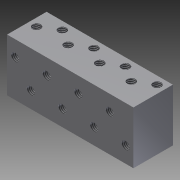
# Autodesk Inventor part: t-manifold ems
Saved by Autodesk Inventor 2011 (Build 150239000, 239)
## iProperties
Created: 2012-03-13
Part Number: t-manifold ems
Document SubType Name: Modeling
Designer: Marc
Density: 1 g/cm^3
Author: Marc
Autodesk Inventor part; units mm, degrees
ref_plane "YZ Plane" through (0, 0, 0) normal (1, 0, 0) x (0, 1, 0)
sketch "Sketch1" plane through (0, 0, 0) normal (0, 0, 1) x (1, 0, 0)
  line L0 (0, 25.4) -> (60.96, 25.4)
  line L1 (60.96, 25.4) -> (60.96, 0)
  line L2 (60.96, 0) -> (0, 0)
  line L3 (0, 0) -> (0, 25.4)
  dimension "tmanifold_width" = 60.96
  dimension "tmanifold_depth" = 25.4
  constraints: 8 end point, 2 parallel, 1 coincident, 1 horizontal, 1 perpendicular
  measures "tmanifold_width" distance of L1.end L2.end
  measures "tmanifold_depth" distance of L0.end L1.end
extrude "Extrusion1" add sketch "Sketch1" along normal blind 19.05
sketch "Sketch2" plane through (0, 0, 19.05) normal (0, 0, 1) x (1, 0, 0)
  line L0 (60.96, 25.4) -> (60.96, 0) projected
  line L1 (0, 25.4) -> (60.96, 25.4) projected
  line L2 (0, 0) -> (0, 25.4) projected
  line L3 (0, 12.7) -> (60.96, 12.7) construction
  line L4 (3.81, 17.78) -> (3.81, 12.7) construction
  line L5 (11.43, 7.62) -> (11.43, 12.7) construction
  point P0 (19.05, 17.78)
  point P1 (26.67, 7.62)
  point P2 (34.29, 17.78)
  point P3 (41.91, 7.62)
  point P4 (49.53, 17.78)
  point P5 (57.15, 7.62)
  dimension "d5" = 7.62
  dimension "d6" = 7.62
  dimension "d9" = 15.24
  dimension "d14" = 3.81
  constraints: 6 end point, 2 midpoint, 2 perpendicular, 2 point on line, 1 horizontal, 1 parallel, 6 other
  measures "d5" horizontal distance of L5.start L4.start
  measures "d6" distance from line of L1 L4.start
  measures "d9" distance of L5.start point (26.67, 7.62)
  measures "d14" distance from line of L2 L4.start
hole "top 10-32 ports" at (3.81, 17.78, 19.05) at (11.43, 7.62, 19.05) at (26.67, 7.62, 19.05) at (19.05, 17.78, 19.05) at (41.91, 7.62, 19.05) at (34.29, 17.78, 19.05) at (57.15, 7.62, 19.05) at (49.53, 17.78, 19.05) direction (0, 0, -1) diameter 3.9624 depth 6.604 thread size "10-32 UNF" class "2B" standard "ANSI Unified Screw Threads"
sketch "Sketch3" plane through (0, 0, 0) normal (0, -1, 0) x (1, 0, 0)
  line L0 (60.96, 19.05) -> (0, 19.05) projected
  line L1 (60.96, 0) -> (0, 0) projected
  line L2 (1.8288, 12.446) -> (1.8288, 19.05) projected
  line L3 (5.7912, 12.446) -> (5.7912, 19.05) projected
  line L4 (5.7912, 12.446) -> (1.8288, 12.446) projected
  line L5 (9.4488, 12.446) -> (9.4488, 19.05) projected
  line L6 (13.4112, 12.446) -> (13.4112, 19.05) projected
  line L7 (13.4112, 12.446) -> (9.4488, 12.446) projected
  line L8 (3.81, 12.446) -> (3.81, 0) construction
  line L9 (11.43, 12.446) -> (11.43, 0) construction
  circle A0 centre (3.81, 8.636) radius 3.81 construction
  circle A1 centre (11.43, 3.81) radius 3.81 construction
  point P0 (19.05, 8.636)
  point P1 (26.67, 3.81)
  point P2 (34.29, 8.636)
  point P3 (41.91, 3.81)
  point P4 (49.53, 8.636)
  point P5 (57.15, 3.81)
  dimension "d22" = 7.62
  dimension "d25" = 15.24
  dimension "d78" = 8.636
  dimension "d79" = 3.81
  constraints: 4 end point, 4 point on line, 2 centre point, 2 coincident, 2 midpoint, 2 perpendicular, 2 tangent, 1 equal radius, 1 horizontal, 6 other
  measures "d22" diameter of A0
  measures "d25" distance of point (3.81, 8.636) point (19.05, 8.636)
  measures "d78" distance from line of L1 point (49.53, 8.636)
  measures "d79" distance from line of L1 point (57.15, 3.81)
hole "front 10-32 ports" at (3.81, 0, 8.636) at (11.43, 0, 3.81) at (19.05, 0, 8.636) at (26.67, 0, 3.81) at (34.29, 0, 8.636) at (41.91, 0, 3.81) at (49.53, 0, 8.636) at (57.15, 0, 3.81) direction (0, 1, 0) diameter 3.9624 depth 6.604 thread size "10-32 UNF" class "2B" standard "ANSI Unified Screw Threads"
sketch "Sketch4" plane through (0, 25.4, 0) normal (0, 1, 0) x (1, 0, 0)
  circle A0 centre (3.81, -8.636) radius 2.5527 projected
  circle A1 centre (11.43, -3.81) radius 2.5527 projected
  circle A2 centre (19.05, -8.636) radius 2.5527 projected
  circle A3 centre (26.67, -3.81) radius 2.5527 projected
  circle A4 centre (34.29, -8.636) radius 2.5527 projected
  circle A5 centre (41.91, -3.81) radius 2.5527 projected
  circle A6 centre (49.53, -8.636) radius 2.5527 projected
  circle A7 centre (57.15, -3.81) radius 2.5527 projected
  dimension "d76" = 4.826
  dimension "d77" = 9.0197
  constraints: 8 coincident
  measures "d76" vertical distance of A7.centre A6.centre
  measures "d77" distance of A6.centre A7.centre
hole "rear 10-32 ports" at (57.15, 25.4, 3.81) at (49.53, 25.4, 8.636) at (41.91, 25.4, 3.81) at (34.29, 25.4, 8.636) at (26.67, 25.4, 3.81) at (19.05, 25.4, 8.636) at (11.43, 25.4, 3.81) at (3.81, 25.4, 8.636) direction (0, -1, 0) diameter 3.9624 depth 6.604 thread size "10-32 UNF" class "2B" standard "ANSI Unified Screw Threads"
sketch "Sketch5" plane through (0, 0, 0) normal (0, -1, 0) x (1, 0, 0)
  circle A0 centre (57.15, 3.81) radius 2.5527 projected
  circle A1 centre (49.53, 8.636) radius 2.5527 projected
  circle A2 centre (41.91, 3.81) radius 2.5527 projected
  circle A3 centre (34.29, 8.636) radius 2.5527 projected
  circle A4 centre (26.67, 3.81) radius 2.5527 projected
  circle A5 centre (19.05, 8.636) radius 2.5527 projected
  circle A6 centre (11.43, 3.81) radius 2.5527 projected
  circle A7 centre (3.81, 8.636) radius 2.5527 projected
  constraints: 8 coincident
hole "air channel thru" at (3.81, 0, 8.636) at (11.43, 0, 3.81) at (19.05, 0, 8.636) at (26.67, 0, 3.81) at (34.29, 0, 8.636) at (41.91, 0, 3.81) at (49.53, 0, 8.636) at (57.15, 0, 3.81) direction (0, 1, 0) diameter 1.016 end through all
sketch "Sketch6" plane through (0, 0, 19.05) normal (0, 0, 1) x (1, 0, 0)
  circle A0 centre (49.53, 17.78) radius 2.5527 projected
  circle A1 centre (57.15, 7.62) radius 2.5527 projected
  circle A2 centre (34.29, 17.78) radius 2.5527 projected
  circle A3 centre (41.91, 7.62) radius 2.5527 projected
  circle A4 centre (19.05, 17.78) radius 2.5527 projected
  circle A5 centre (26.67, 7.62) radius 2.5527 projected
  circle A6 centre (11.43, 7.62) radius 2.5527 projected
  circle A7 centre (3.81, 17.78) radius 2.5527 projected
  constraints: 8 coincident
ref_plane "Work Plane1" through (3.81, 0, 8.636) normal (0, 0, 1) x (1, 0, 0)
ref_plane "Work Plane2" through (11.43, 0, 3.81) normal (0, 0, 1) x (1, 0, 0)
hole "Hole5" at (3.81, 17.78, 19.05) at (19.05, 17.78, 19.05) at (34.29, 17.78, 19.05) at (49.53, 17.78, 19.05) direction (0, 0, -1) diameter 1.016 depth 10.414
hole "Hole6" at (11.43, 7.62, 19.05) at (26.67, 7.62, 19.05) at (41.91, 7.62, 19.05) at (57.15, 7.62, 19.05) direction (0, 0, -1) diameter 1.016 depth 15.24
sketch "Sketch7" plane through (0, 0, 0) normal (0, 0, -1) x (-1, 0, 0)
  line L0 (-1.8288, 6.604) -> (-1.8288, 0) projected
  line L1 (-5.7912, 6.604) -> (-5.7912, 0) projected
  line L2 (-3.302, 18.796) -> (-3.302, 6.604) projected
  line L3 (-4.318, 18.796) -> (-4.318, 6.604) projected
  line L4 (-1.8288, 18.796) -> (-1.8288, 25.4) projected
  line L5 (-5.7912, 18.796) -> (-5.7912, 25.4) projected
  line L6 (-1.8288, 18.796) -> (-5.7912, 18.796) projected
  line L7 (-5.7912, 6.604) -> (-1.8288, 6.604) projected
  line L8 (-8.8773, 0) -> (-13.9827, 0) projected
  line L9 (-13.4112, 0.5715) -> (-9.4488, 0.5715) projected
  line L10 (-13.4112, 6.604) -> (-13.4112, 0) projected
  line L11 (-9.4488, 6.604) -> (-9.4488, 0) projected
  line L12 (-10.922, 18.796) -> (-10.922, 6.604) projected
  line L13 (-11.938, 18.796) -> (-11.938, 6.604) projected
  line L14 (-9.4488, 18.796) -> (-13.4112, 18.796) projected
  line L15 (-18.542, 18.796) -> (-18.542, 6.604) projected
  line L16 (-19.558, 18.796) -> (-19.558, 6.604) projected
  line L17 (-21.0312, 6.604) -> (-17.0688, 6.604) projected
  line L18 (-28.6512, 6.604) -> (-24.6888, 6.604) projected
  line L19 (-36.2712, 6.604) -> (-32.3088, 6.604) projected
  line L20 (-31.7373, 0) -> (-36.8427, 0) projected
  line L21 (-43.8912, 6.604) -> (-39.9288, 6.604) projected
  line L22 (-51.5112, 6.604) -> (-47.5488, 6.604) projected
  line L23 (-49.022, 18.796) -> (-49.022, 6.604) projected
  line L24 (-50.038, 18.796) -> (-50.038, 6.604) projected
  line L25 (-49.022, 18.796) -> (-49.022, 6.604) projected
  line L26 (-50.038, 18.796) -> (-50.038, 6.604) projected
  line L27 (-33.782, 18.796) -> (-33.782, 6.604) projected
  line L28 (-33.782, 18.796) -> (-33.782, 6.604) projected
  line L29 (-32.3088, 6.604) -> (-32.3088, 0) projected
  line L30 (-33.782, 18.796) -> (-33.782, 6.604) projected
  line L31 (-33.782, 18.796) -> (-33.782, 6.604) projected
  line L32 (-41.402, 18.796) -> (-41.402, 6.604) projected
  line L33 (-42.418, 18.796) -> (-42.418, 6.604) projected
  line L34 (-27.178, 18.796) -> (-27.178, 6.604) projected
  line L35 (-21.0312, 18.796) -> (-21.0312, 25.4) projected
  line L36 (-27.178, 18.796) -> (-27.178, 6.604) projected
  line L37 (-42.418, 18.796) -> (-42.418, 6.604) projected
  line L38 (-36.2712, 18.796) -> (-36.2712, 25.4) projected
  line L39 (-34.798, 18.796) -> (-34.798, 6.604) projected
  line L40 (-39.9288, 18.796) -> (-43.8912, 18.796) projected
  line L41 (-47.5488, 18.796) -> (-51.5112, 18.796) projected
  line L42 (-55.1688, 18.796) -> (-59.1312, 18.796) projected
  line L43 (-56.642, 18.796) -> (-56.642, 6.604) projected
  line L44 (-57.658, 18.796) -> (-57.658, 6.604) projected
  line L45 (-59.1312, 6.604) -> (-55.1688, 6.604) projected
  line L46 (-32.3088, 18.796) -> (-36.2712, 18.796) projected
  line L47 (-26.162, 18.796) -> (-26.162, 6.604) projected
  line L48 (-24.6888, 18.796) -> (-28.6512, 18.796) projected
  line L49 (-60.96, 25.4) -> (-60.96, 0) projected
  line L50 (0, 25.4) -> (-60.96, 25.4) projected
  line L51 (0, 0) -> (0, 25.4) projected
  line L52 (-60.96, 0) -> (0, 0) projected
  line L53 (-28.6512, 6.604) -> (-28.6512, 0) projected
  line L54 (-24.6888, 6.604) -> (-24.6888, 0) projected
  line L55 (-36.2712, 6.604) -> (-36.2712, 0) projected
  line L56 (-39.9288, 6.604) -> (-39.9288, 0) projected
  line L57 (-43.8912, 6.604) -> (-43.8912, 0) projected
  line L58 (-47.5488, 6.604) -> (-47.5488, 0) projected
  line L59 (-51.5112, 6.604) -> (-51.5112, 0) projected
  line L60 (-55.1688, 6.604) -> (-55.1688, 0) projected
  line L61 (-59.1312, 6.604) -> (-59.1312, 0) projected
  line L62 (-39.9288, 18.796) -> (-39.9288, 25.4) projected
  line L63 (-43.8912, 18.796) -> (-43.8912, 25.4) projected
  line L64 (-51.5112, 18.796) -> (-51.5112, 25.4) projected
  line L65 (-55.1688, 18.796) -> (-55.1688, 25.4) projected
  line L66 (-59.1312, 18.796) -> (-59.1312, 25.4) projected
  line L67 (-17.0688, 18.796) -> (-21.0312, 18.796) projected
  line L68 (-17.0688, 18.796) -> (-17.0688, 25.4) projected
  line L69 (-17.0688, 6.604) -> (-17.0688, 0) projected
  line L70 (-21.0312, 6.604) -> (-21.0312, 0) projected
  line L71 (-13.4112, 18.796) -> (-13.4112, 25.4) projected
  line L72 (-9.4488, 18.796) -> (-9.4488, 25.4) projected
  circle A0 centre (-34.29, 17.78) radius 2.5527 projected
  circle A1 centre (-19.05, 17.78) radius 2.5527 projected
  circle A2 centre (-3.81, 17.78) radius 2.5527 projected
  circle A3 centre (-11.43, 7.62) radius 2.5527 projected
  circle A4 centre (-26.67, 7.62) radius 2.5527 projected
  circle A5 centre (-41.91, 7.62) radius 2.5527 projected
  circle A6 centre (-49.53, 17.78) radius 2.5527 projected
  circle A7 centre (-57.15, 7.62) radius 2.5527 projected
  line L73 (-32.3088, 18.796) -> (-32.3088, 25.4) projected
  line L74 (-28.6512, 18.796) -> (-28.6512, 25.4) projected
  line L75 (-24.6888, 18.796) -> (-24.6888, 25.4) projected
  line L76 (-13.4112, 6.604) -> (-9.4488, 6.604) projected
  line L77 (-47.5488, 18.796) -> (-47.5488, 25.4) projected
  line L78 (-60.96, 12.7) -> (0, 12.7) construction
  line L79 (-30.48, 25.4) -> (-30.48, 0) construction
  point P0 (-9.4488, 0.5715)
  point P1 (-30.48, 12.7)
  point P2 (-15.24, 12.7)
  point P3 (-45.72, 12.7)
  dimension "d68" = 15.24
  constraints: 5 midpoint, 4 end point, 1 point on line, 1 symmetric about line, 2 other
  measures "d68" distance of point (-30.48, 12.7) point (-15.24, 12.7)
sketch "Sketch8" plane through (0, 0, 19.05) normal (0, 0, 1) x (1, 0, 0)
  circle A0 centre (49.53, 17.78) radius 2.5527 projected
  circle A1 centre (57.15, 7.62) radius 2.5527 projected
  circle A2 centre (34.29, 17.78) radius 2.5527 projected
  circle A3 centre (41.91, 7.62) radius 2.5527 projected
  circle A4 centre (19.05, 17.78) radius 2.5527 projected
  circle A5 centre (26.67, 7.62) radius 2.5527 projected
  circle A6 centre (11.43, 7.62) radius 2.5527 projected
  circle A7 centre (3.81, 17.78) radius 2.5527 projected
  line L0 (60.96, 25.4) -> (60.96, 0) projected
  line L1 (0, 25.4) -> (60.96, 25.4) projected
  line L2 (0, 0) -> (0, 25.4) projected
  line L3 (60.96, 0) -> (0, 0) projected
  line L4 (0, 12.7) -> (60.96, 12.7) construction
  line L5 (0, 12.7) -> (60.96, 12.7)
  line L6 (30.48, 0) -> (30.48, 25.4) construction
  line L7 (11.938, 18.796) -> (11.938, 6.604) projected
  line L8 (10.922, 18.796) -> (10.922, 6.604) projected
  line L9 (18.542, 18.796) -> (18.542, 6.604) projected
  line L10 (19.558, 18.796) -> (19.558, 6.604) projected
  line L11 (26.162, 18.796) -> (26.162, 6.604) projected
  line L12 (27.178, 18.796) -> (27.178, 6.604) projected
  line L13 (33.782, 18.796) -> (33.782, 6.604) projected
  line L14 (34.798, 18.796) -> (34.798, 6.604) projected
  line L15 (42.418, 18.796) -> (42.418, 6.604) projected
  line L16 (41.402, 18.796) -> (41.402, 6.604) projected
  line L17 (49.022, 18.796) -> (49.022, 6.604) projected
  line L18 (50.038, 18.796) -> (50.038, 6.604) projected
  point P0 (30.48, 12.7)
  point P1 (45.72, 12.7)
  point P2 (15.24, 12.7)
  dimension "d66" = 30.48
  dimension "d67" = 15.24
  constraints: 6 end point, 5 midpoint, 2 point on line, 1 perpendicular, 1 symmetric about line
  measures "d66" distance of L0.start L6.end
  measures "d67" distance of point (45.72, 12.7) point (30.48, 12.7)
hole "Hole7" at (30.48, 12.7, 0) at (15.24, 12.7, 0) at (45.72, 12.7, 0) direction (0, 0, 1) diameter 3.302 depth 12.7 tip angle 118 thread size "8-32 UNC" class "2B" standard "ANSI Unified Screw Threads"
body "Solid1"
